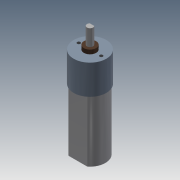
# Autodesk Inventor part: dc-motor_12V_60U-min
Saved by Autodesk Inventor 2018 (Build 220112000, 112)
## iProperties
Created: 2013-12-18
Part Number: dc-motor_12V_60U-min
Material: Aluminium 6061
Document SubType Name: Modeling
Designer: 4ndreas
Density: 2.71 g/cm^3
Appearance: Stahl
Mass: 20.9269 g
Surface Area: 26.1787 cm^2
Volume: 7.72211 cm^3
Author: 4ndreas
Autodesk Inventor part; units mm, degrees
ref_plane "YZ Plane" through (0, 0, 0) normal (1, 0, 0) x (0, 1, 0)
ref_plane "XZ Plane" through (0, 0, 0) normal (0, 1, 0) x (-1, 0, 0)
ref_plane "XY Plane" through (0, 0, 0) normal (0, 0, 1) x (1, 0, 0)
sketch "Skizze1" plane through (0, 0, 0) normal (0, 0, 1) x (1, 0, 0)
  circle A0 centre (0, 0) radius 8
  line L0 (-5.5, 0) -> (5.5, 0) construction
  circle A1 centre (0, 0) radius 3
  circle A2 centre (0, 0) radius 1.5
  arc A3 (-1.118, 1) -> (1.118, 1) centre (0, 0) ccw construction
  line L1 (-1.118, 1) -> (1.118, 1)
  dimension "d3" = 3
  dimension "d0" = 16
  dimension "d1" = 11
  dimension "d2" = 6
  dimension "d4" = 2.5
  constraints: 5 coincident, 4 end point, 3 centre point, 2 point on circle, 1 horizontal, 1 midpoint, 1 parallel, 4 other
  measures "d0" diameter of A0
  measures "d1" distance of L0.start L0.end
  measures "d2" diameter of A1
extrude "Extrusion1" add sketch "Skizze1" along normal blind 2 contours A1 | A2 L1 | L1 A2
sketch "Skizze2" plane through (0, 0, 2) normal (0, 0, 1) x (1, 0, 0)
  circle A0 centre (0, 0) radius 1.5 projected
extrude "Extrusion2" add sketch "Skizze2" along normal blind 1
sketch "Skizze3" plane through (0, 0, 3) normal (0, 0, 1) x (1, 0, 0)
  circle A0 centre (0, 0) radius 1.5 projected
  line L0 (-1.118, 1) -> (1.118, 1) projected
  circle A1 centre (0, 0) radius 1.5 projected
extrude "Extrusion3" add sketch "Skizze3" along normal blind 7 contours A0 L0 picked at (0.0594, 0.1702)
extrude "Extrusion4" add sketch "Skizze1" against normal blind 14.5 contours A0 | A1 | A2 L1 | L1 A2
sketch "Skizze4" plane through (0, 0, -14.5) normal (0, 0, -1) x (-1, 0, 0)
  circle A0 centre (0, 0) radius 8 projected
  arc A1 (-4.5983, 5.925) -> (-4.5983, -5.925) centre (0, 0) ccw
  arc A2 (4.5983, -5.925) -> (4.5983, 5.925) centre (0, 0) ccw
  line L0 (-4.5983, 5.925) -> (4.5983, 5.925)
  line L1 (4.5983, -5.925) -> (-4.5983, -5.925)
  dimension "d14" = 7.5
  dimension "d15" = 11.85
  constraints: 4 end point, 4 point on circle, 2 centre point, 2 coincident, 2 parallel, 1 concentric, 1 horizontal
  measures "d14" radius of A1
  measures "d15" distance between parallel lines of L1 L0
extrude "Extrusion5" add sketch "Skizze4" along normal blind 30 contours L0 A2 L1 A1
hole "Bohrung1" at (-5.5, 0, 0) at (5.5, 0, 0) direction (0, 0, -1) diameter 1.567 depth 3 tip angle 118 thread size "M2x0.4" class "6H" standard "ANSI Metric M Profile"
